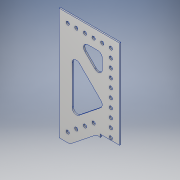
# Autodesk Inventor part: SUP_017_CutNewerTop4BarBarGusset
Saved by Autodesk Inventor 2018.3 (Build 223284000, 284)
## iProperties
Created: 2020-02-11
Part Number: SUP_017_CutNewerTop4BarBarGusset
Material: Aluminum 6061
Document SubType Name: Modeling
Designer: 22barlalex
Density: 2.7 g/cm^3
Appearance: Aluminum - Flat
Author: 22barlalex
Autodesk Inventor part; units mm, degrees
ref_plane "YZ Plane" through (0, 0, 0) normal (1, 0, 0) x (0, 1, 0)
ref_plane "XZ Plane" through (0, 0, 0) normal (0, 1, 0) x (-1, 0, 0)
ref_plane "XY Plane" through (0, 0, 0) normal (0, 0, 1) x (1, 0, 0)
sketch "Sketch1" plane through (0, 0, 0) normal (0, 0, 1) x (1, 0, 0)
  line L0 (0, 0) -> (0, -165.1)
  line L1 (0, -165.1) -> (-25.4, -165.1)
  line L2 (-25.4, -165.1) -> (-25.4, -127)
  line L3 (-25.4, -127) -> (-72.973588, -165.1)
  line L4 (-72.973588, -165.1) -> (-88.851291, -145.274296)
  line L5 (-25.4, -94.458406) -> (-25.4, -25.4)
  line L6 (-25.4, -25.4) -> (-88.9, -25.4)
  line L7 (-88.9, -25.4) -> (-88.9, 0)
  line L8 (-88.9, 0) -> (0, 0)
  line L9 (-88.9, 0) -> (-88.9, -189.087308) construction
  line L10 (-121.475506, -165.1) -> (0, -165.1) construction
  line L11 (-88.851291, -145.274296) -> (-25.4, -94.458406)
  dimension "d0" = 165.1
  dimension "d1" = 25.4
  dimension "d2" = 38.1
  dimension "d3" = 25.4
  dimension "d4" = 25.4
  dimension "d5" = 88.9
  dimension "d6" = 51.31
  constraints: 24 end point, 7 perpendicular, 3 point on line, 2 vertical, 1 parallel
  measures "d0" distance of L0.start L0.end
  measures "d1" distance of L0.end L1.end
  measures "d2" distance of L1.end L2.end
  measures "d3" distance of L4.end L3.end
  measures "d4" distance between parallel lines of L8 L6
  measures "d5" distance between parallel lines of L0 L7
  measures "d6" angle of L2 L3
sketch "Sketch1 outline for Extrusion1" plane through (0, 0, 0) normal (0, 0, 1) x (1, 0, 0)
  line L0 (0, 0) -> (0, -165.1)
  line L1 (0, -165.1) -> (-25.4, -165.1)
  line L2 (-25.4, -165.1) -> (-25.4, -127)
  line L3 (-25.4, -127) -> (-72.973588, -165.1)
  line L4 (-72.973588, -165.1) -> (-88.851291, -145.274296)
  line L5 (-88.851291, -145.274296) -> (-25.4, -94.458406)
  line L6 (-25.4, -94.458406) -> (-25.4, -25.4)
  line L7 (-25.4, -25.4) -> (-88.9, -25.4)
  line L8 (-88.9, -25.4) -> (-88.9, 0)
  line L9 (-88.9, 0) -> (0, 0)
extrude "Extrusion1" add sketch "Sketch1 outline for Extrusion1" along normal blind 2.032
sketch "Sketch2" plane through (0, 0, 2.032) normal (0, 0, 1) x (1, 0, 0)
  line L0 (-88.9, -25.4) -> (-25.4, -25.4)
  line L1 (-88.9, -25.4) -> (-25.4, -88.9)
  line L2 (-88.9, -25.4) -> (0.902561, -25.4) construction
  line L3 (-61.959232, -25.4) -> (-25.4, -61.959232)
  line L4 (-25.4, -61.959232) -> (-25.4, -88.9)
  line L5 (-25.4, -88.9) -> (-25.4, -61.959232)
  line L6 (-61.959232, -25.4) -> (-88.9, -25.4)
  line L7 (-88.9, -145.213476) -> (-88.9, -25.4)
  line L8 (-69.85, -130.056836) -> (-69.85, -44.45)
  line L9 (-25.4, -88.9) -> (-88.9, -25.4)
  line L10 (-25.4, -25.4) -> (-88.9, -25.4)
  line L11 (-88.9, -25.4) -> (-61.959232, -25.4)
  line L12 (-61.959232, -25.4) -> (-25.4, -61.959232)
  line L13 (-25.4, -61.959232) -> (-25.4, -88.9)
  line L14 (-25.4, -88.9) -> (-25.4, -61.959232)
  line L15 (-25.4, -88.9) -> (-25.4, -61.959232)
  line L16 (-88.9, -145.213476) -> (-88.9, -165.1)
  line L17 (-72.973588, -165.1) -> (-25.4, -127)
  line L18 (-49.186794, -146.05) -> (-25.4, -146.05)
  line L19 (-25.4, -127) -> (-25.4, -165.1)
  line L20 (-72.973588, -165.1) -> (-49.186794, -146.05)
  line L21 (-88.851291, -145.274296) -> (-72.973588, -165.1)
  line L22 (-25.4, -146.05) -> (-25.4, -165.1)
  line L23 (-88.9, -165.1) -> (-25.4, -165.1)
  line L24 (-88.9, 0) -> (-88.9, -25.4)
  line L25 (-72.973588, -165.1) -> (-88.851291, -145.274296)
  line L26 (-88.851291, -145.274296) -> (-69.85, -130.056836)
  line L27 (-25.4, -94.458406) -> (-88.851291, -145.274296)
  line L28 (-49.186794, -146.05) -> (-25.4, -146.05)
  line L29 (-25.4, -165.1) -> (-25.4, -146.05)
  line L30 (-25.4, -165.1) -> (-72.973588, -165.1)
  line L31 (-72.973588, -165.1) -> (-88.9, -165.1)
  line L32 (-88.9, -165.1) -> (-88.9, -25.4)
  point P0 (0, 0)
  dimension "d10" = 45
  dimension "d11" = 19.05
  dimension "d12" = 19.05
  dimension "d16" = 19.05
  constraints: 52 end point, 16 collinear, 3 horizontal, 3 point on line, 3 vertical, 2 midpoint, 2 parallel, 1 equal length
  measures "d10" angle of L1 L2
  measures "d11" distance between parallel lines of L3 L1
  measures "d12" distance between parallel lines of L7 L8
  measures "d16" distance between parallel lines of L23 L18
sketch "Sketch2 outline for Extrusion3" plane through (0, 0, 2.032) normal (0, 0, 1) x (1, 0, 0)
  line L0 (-49.186794, -146.05) -> (-72.973588, -165.1)
  line L1 (-25.4, -146.05) -> (-49.186794, -146.05)
  line L2 (-25.4, -165.1) -> (-25.4, -146.05)
  line L3 (-72.973588, -165.1) -> (-25.4, -165.1)
  line L4 (-61.959232, -25.4) -> (-25.4, -61.959232)
  line L5 (-25.4, -61.959232) -> (-25.4, -88.9)
  line L6 (-25.4, -88.9) -> (-69.85, -44.45)
  line L7 (-69.85, -44.45) -> (-69.85, -130.056836)
  line L8 (-69.85, -130.056836) -> (-88.851291, -145.274296)
  line L9 (-88.851291, -145.274296) -> (-72.973588, -165.1)
  line L10 (-72.973588, -165.1) -> (-88.9, -165.1)
  line L11 (-88.9, -165.1) -> (-88.9, -25.4)
  line L12 (-88.9, -25.4) -> (-61.959232, -25.4)
extrude "Extrusion3" add sketch "Sketch2 outline for Extrusion3" against normal blind 2.032
sketch "Sketch3" plane through (0, 0, 2.032) normal (0, 0, 1) x (1, 0, 0)
  line L0 (0, 0) -> (-88.9, 0)
  line L1 (0, -165.1) -> (0, 0)
  line L2 (0, -90.387243) -> (-102.323642, -172.334622) construction
  line L3 (-25.4, -94.458406) -> (-69.85, -130.056836) construction
  point P0 (-63.5, -12.7)
  point P1 (-50.8, -12.7)
  point P2 (-38.1, -12.7)
  point P3 (-25.4, -12.7)
  point P4 (-12.7, -12.7)
  point P5 (-12.7, -25.4)
  point P6 (-12.7, -38.1)
  point P7 (-12.7, -50.8)
  point P8 (-12.7, -63.5)
  point P9 (-12.7, -76.2)
  point P10 (-12.7, -88.9)
  point P11 (-12.7, -101.6)
  point P12 (-38.1, -120.900183)
  point P13 (-50.8, -131.071163)
  point P14 (-63.5, -141.242143)
  point P15 (-76.2, -151.413123)
  point P16 (-76.2, -12.7)
  point P17 (-12.7, -114.3)
  point P18 (-12.7, -127)
  point P19 (-12.7, -139.7)
  point P20 (-12.7, -152.4)
  dimension "d19" = 12.7
  dimension "d20" = 12.7
  dimension "d21" = 12.7
  dimension "d22" = 12.7
  dimension "d23" = 12.7
  dimension "d24" = 12.7
  dimension "d25" = 12.7
  dimension "d26" = 12.7
  dimension "d27" = 12.7
  dimension "d28" = 12.7
  dimension "d29" = 12.7
  dimension "d30" = 12.7
  dimension "d31" = 12.7
  dimension "d32" = 12.7
  dimension "d33" = 12.7
  dimension "d34" = 12.7
  dimension "d35" = 12.7
  dimension "d37" = 12.7
  dimension "d39" = 12.7
  dimension "d40" = 38.1
  dimension "d41" = 50.8
  dimension "d42" = 63.5
  dimension "d43" = 76.2
  constraints: 11 vertical alignment, 5 horizontal alignment, 5 point on line, 2 end point
  measures "d19" distance from line of L0 point (-12.7, -12.7)
  measures "d20" distance of point (-12.7, -12.7) point (-12.7, -25.4)
  measures "d21" distance of point (-12.7, -25.4) point (-12.7, -38.1)
  measures "d22" distance of point (-12.7, -38.1) point (-12.7, -50.8)
  measures "d23" distance of point (-12.7, -50.8) point (-12.7, -63.5)
  measures "d24" distance of point (-12.7, -63.5) point (-12.7, -76.2)
  measures "d25" distance of point (-12.7, -76.2) point (-12.7, -88.9)
  measures "d26" distance of point (-12.7, -88.9) point (-12.7, -101.6)
  measures "d27" distance of point (-12.7, -12.7) point (-25.4, -12.7)
  measures "d28" distance of point (-38.1, -12.7) point (-25.4, -12.7)
  measures "d29" distance of point (-38.1, -12.7) point (-50.8, -12.7)
  measures "d30" distance of point (-50.8, -12.7) point (-63.5, -12.7)
  measures "d31" distance of point (-63.5, -12.7) point (-76.2, -12.7)
  measures "d32" distance of point (-12.7, -101.6) point (-12.7, -114.3)
  measures "d33" distance of point (-12.7, -114.3) point (-12.7, -127)
  measures "d34" distance of point (-12.7, -127) point (-12.7, -139.7)
  measures "d35" distance of point (-12.7, -139.7) point (-12.7, -152.4)
  measures "d37" distance from line of L1 point (-12.7, -12.7)
  measures "d39" distance between parallel lines of L3 L2
  measures "d40" distance from line of L1 point (-38.1, -120.9)
  measures "d41" distance from line of L1 point (-50.8, -131.071)
  measures "d42" distance from line of L1 point (-63.5, -141.242)
  measures "d43" distance from line of L1 point (-76.2, -151.413)
hole "Hole1" at (-63.5, -12.7, 2.032) at (-50.8, -12.7, 2.032) at (-38.1, -12.7, 2.032) at (-25.4, -12.7, 2.032) at (-12.7, -12.7, 2.032) at (-12.7, -25.4, 2.032) at (-12.7, -38.1, 2.032) at (-12.7, -50.8, 2.032) at (-12.7, -63.5, 2.032) at (-12.7, -76.2, 2.032) at (-12.7, -88.9, 2.032) at (-12.7, -101.6, 2.032) at (-38.1, -120.900183, 2.032) at (-50.8, -131.071163, 2.032) at (-63.5, -141.242143, 2.032) at (-76.2, -151.413123, 2.032) at (-76.2, -12.7, 2.032) at (-12.7, -114.3, 2.032) at (-12.7, -127, 2.032) at (-12.7, -139.7, 2.032) at (-12.7, -152.4, 2.032) direction (0, 0, -1) diameter 4.8514 end through all
fillet "Fillet1" radius 6.35 4 edges at (-25.4, -94.4584, 1.016) (-25.4, -88.9, 1.016) (-69.85, -44.45, 1.016) (-69.85, -130.0568, 1.016)
fillet "Fillet4" radius 6.35 3 edges at (-25.4, -25.4, 1.016) (-61.9592, -25.4, 1.016) (-25.4, -61.9592, 1.016)
sketch "Sketch5" plane through (0, 0, 2.032) normal (0, 0, 1) x (1, 0, 0)
  line L0 (-49.186794, -146.05) -> (-25.4, -127)
  line L1 (-49.186794, -146.05) -> (-25.4, -146.05)
  line L2 (-25.4, -146.05) -> (-25.4, -127)
  line L3 (-49.186794, -146.05) -> (-25.4, -146.05)
  line L4 (-25.4, -127) -> (-49.186794, -146.05)
  point P0 (0, 0)
  constraints: 6 end point, 1 horizontal, 1 perpendicular
sketch "Sketch5 outline for Extrusion5" plane through (0, 0, 2.032) normal (0, 0, 1) x (1, 0, 0)
  line L0 (-49.186794, -146.05) -> (-25.4, -127)
  line L1 (-25.4, -127) -> (-25.4, -146.05)
  line L2 (-25.4, -146.05) -> (-49.186794, -146.05)
extrude "Extrusion5" add sketch "Sketch5 outline for Extrusion5" against normal blind 2.032
sketch "Sketch6" plane through (0, 0, 2.032) normal (0, 0, 1) x (1, 0, 0)
  line L0 (0, -165.1) -> (-88.9, -165.1)
  line L1 (-72.973588, -165.1) -> (-25.4, -127)
  line L2 (-25.4, -127) -> (-25.4, -165.1)
  line L3 (0, -165.1) -> (0, 0)
  line L4 (-27.848185, -96.419071) -> (-59.530574, -121.792373)
  line L5 (-72.973588, -165.1) -> (-25.4, -165.1)
  dimension "d59" = 25.4
  dimension "d60" = 25.4
  constraints: 6 end point, 2 parallel, 2 point on line, 1 collinear, 1 vertical
  measures "d59" distance between parallel lines of L4 L1
  measures "d60" distance between parallel lines of L3 L2
sketch "Sketch6 outline for Extrusion6" plane through (0, 0, 2.032) normal (0, 0, 1) x (1, 0, 0)
  line L0 (-25.4, -127) -> (-72.973588, -165.1)
  line L1 (-25.4, -165.1) -> (-25.4, -127)
  line L2 (-72.973588, -165.1) -> (-25.4, -165.1)
extrude "Extrusion6" cut sketch "Sketch6 outline for Extrusion6" against normal blind 2.032
fillet "Fillet5" radius 6.35 1 edges at (-25.4, -127, 1.016)
sketch "Sketch7" plane through (0, -165.1, 0) normal (0, -1, 0) x (1, 0, 0)
  line L0 (-88.9, 0) -> (0, 0)
  line L1 (-25.4, 2.032) -> (-35.719426, 2.032)
  line L2 (0, 0) -> (-28.56159, 0)
  line L3 (-28.56159, 0) -> (-28.56159, 2.032)
  line L4 (-28.56159, 2.032) -> (0, 2.032)
  line L5 (0, 2.032) -> (0, 0)
  constraints: 8 end point, 2 parallel, 1 horizontal, 1 perpendicular, 1 point on line
sketch "Sketch7 outline for Extrusion7" plane through (0, -165.1, 0) normal (0, -1, 0) x (1, 0, 0)
  line L0 (0, 0) -> (-28.56159, 0)
  line L1 (-28.56159, 0) -> (-28.56159, 2.032)
  line L2 (-28.56159, 2.032) -> (0, 2.032)
  line L3 (0, 2.032) -> (0, 0)
extrude "Extrusion7" cut sketch "Sketch7 outline for Extrusion7" against normal blind 34.925
equation "\"d20\" = d19"
equation "\"d21\" = d19"
equation "\"d22\" = d19"
equation "\"d23\" = d19"
equation "\"d24\" = d19"
equation "\"d25\" = d19"
equation "\"d26\" = d19"
equation "\"d28\" = d27"
equation "\"d29\" = d27"
equation "\"d30\" = d27"
equation "\"d31\" = d27"
equation "\"d32\" = d19"
equation "\"d33\" = d19"
equation "\"d34\" = d19"
equation "\"d35\" = d19"
body "Solid1"
